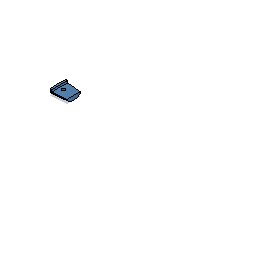
Limiter1 (Autodesk Fusion 360 design; units mm, degrees)
Autodesk Fusion 360 part; units mm, degrees
sketch "Sketch1" plane through (0, -29, 0) normal (0, -1, 0) x (1, 0, 0)
  circle A0 centre (0, 0) radius 92
  circle A1 centre (0, 0) radius 76.573
  arc A2 (-77.2778, 6.7609) -> (-77.2778, -6.7609) centre (0, 0) ccw
  line L0 (0, 0) -> (-106.9698, 0) construction
  line L1 (-77.2778, 6.7609) -> (-91.6499, 8.0183)
  line L2 (-77.2778, -6.7609) -> (-91.6499, -8.0183)
  circle A3 centre (-88, 0) radius 1.7
  dimension "d694" = 1
  dimension "d695" = 88
  dimension "d696" = 3.4
  dimension "d697" = 10
  constraint coincident A0.centre A1.centre
  constraint horizontal L0
  constraint coincident A0 L1.end
  constraint coincident A0 L2.end
  constraint coincident A0.centre L1
  constraint coincident A0.centre L2
  constraint symmetric L0 L1 L2
  constraint coincident L0 A3.centre
  measures "d694" distance of A1 A2
  measures "d695" distance of A0.centre A3.centre
  measures "d696" diameter of A3
  measures "d697" angle of L1 L2
extrude "Extrude1" add sketch "Sketch1" along normal blind 4 contours A0 A2 L1 L2 picked at (-85.4355, -5.4539)
chamfer "Chamfer1" distance 1.55 angle 45 1 edges at (-89.585, -33, 0.6147)
sketch "Sketch2" plane through (0, -33, 0) normal (0, -1, 0) x (1, 0, 0)
  line L0 (-77.2778, 6.7609) -> (-91.6499, 8.0183)
  arc A0 (-91.6499, 8.0183) -> (-91.6499, -8.0183) centre (0, 0) ccw
  line L1 (-91.6499, -8.0183) -> (-77.2778, -6.7609)
  arc A1 (-77.2778, 6.7609) -> (-77.2778, -6.7609) centre (0, 0) ccw
  circle A2 centre (-88, 0) radius 3.25
  arc A3 (-93.6423, 8.1926) -> (-93.6423, -8.1926) centre (0, 0) ccw
  line L2 (-91.6499, 8.0183) -> (-93.6423, 8.1926)
  line L3 (-91.6499, -8.0183) -> (-93.6423, -8.1926)
  dimension "d701" = 2
  constraint coincident A0.centre A1.centre
  constraint coincident L0.end A0.start
  constraint coincident A0.end L1.start
  constraint coincident L0 A3.start
  constraint coincident L1 A3.end
  measures "d701" distance of A0 A3
extrude "Extrude2" add sketch "Sketch2" against normal blind 6 contours A0 A3 L2 L3
chamfer "Chamfer2" distance 3 angle 45 2 edges at (-85.4601, -33, -7.4768) (-85.4601, -33, 7.4768)
fillet "Fillet2" radius 1 2 edges at (-93.6423, -28.5, 8.1926) (-93.6423, -28.5, -8.1926)
